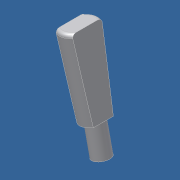
# Autodesk Inventor part: M20E-toggles
Saved by Autodesk Inventor 2015 SP1 (Build 190203100, 203)
## iProperties
Category: PARTsolutions
Created: 2013-12-29
Part Number: M20E-toggles
Catalog Web Link: www.cadenas.de
Description: Bushing Mount Miniature Toggles - toggles - Series M - Miniature Toggles
Document SubType Name: Modeling
Designer: PARTsolutions
Material: Generic
Density: 1 g/cm^3
Appearance: RGB(192,192,192)
NB: M20E-toggles
NN: Bushing Mount Miniature Toggles - toggles
NT: Series M - Miniature Toggles
NBSYN: $PN.-toggles
LINA: M20E-toggles
PN: M20E
SRS: M20
TGGLSALG: 'S', 'S - .413" (10.5mm) Bat','S2', 'S2 - .200" (5.08mm) Bat','S3', 'S3 - .256" (6.5mm) Bat','E', 'E - .450" (11.4mm) Flatted','E2', 'E2 - .256" (6.5mm) Flatted','E4', 'E4 - .840" (21.3mm) Flatted','Q', 'Q - .550" (14.0mm) Cone','Q2', 'Q2 - .640" (16.26mm) Cone','Q4', 'Q4 - .840" (21.3mm) Cone','C', 'C - .571" (14.5mm) Color Tipped Cone','D', 'D - .840" (21.3mm) Color Tipped Cone','K1', 'K1 - .370" (9.4mm) Paddle','K2', 'K2 - .559" (14.2mm) Paddle','B', 'B - .453" (11.5mm) Large Bat','B2', 'B2 - .689" (17.5mm) Large Bat','R', 'R - .610" (15.5mm) Large Flatted','L', 'L - .201" (5.1mm) Dia. Locking Lever'
TGGLS: E
CPSALG: '','N/A'
CCLRALG: '','N/A'
HEIGHT: 0.450
SHEIGHT: 0.087
ROTALG: 0.350
CPCAP: 0.000
KT: DUMMY
SUPPLIER: NKKSWITCHES
ARTICLENO: M20E-toggles
BOMINFO: M20E-toggles
CREATOR: CADENAS GmbH
PSOL_IDENT_0: {$CADENAS_DATA\23d-libs\nkkswitches\toggle\m\parts\m_bt_toggle.prj},215 {VTYP=3D},{NB=M20E-toggles},
PSOL_IDENT_1: {LINA=M20E-toggles},{NN=Bushing Mount Miniature Toggles - toggles},{DATE=28.05.2013 12:02:29},{GEOMD
PSOL_IDENT_2: ATE=28.05.2013 14:02:00},{VERSION=},{LINEID=10},{LINESUBID=-1},{WBVAR=TGGLS,CPS,CCLR}  {NB=M20E-togg
PSOL_IDENT_3: les},{LINA=M20E-toggles},{KT=DUMMY},{PN=M20E},{SRS=M20},{TGGLSALG='S', 'S - .413\" (10.5mm) Bat','S2
PSOL_IDENT_4: ', 'S2 - .200\" (5.08mm) Bat','S3', 'S3 - .256\" (6.5mm) Bat','E', 'E - .450\" (11.4mm) Flatted','E2
PSOL_IDENT_5: ', 'E2 - .256\" (6.5mm) Flatted','E4', 'E4 - .840\" (21.3mm) Flatted','Q', 'Q - .550\" (14.0mm) Cone
PSOL_IDENT_6: ','Q2', 'Q2 - .640\" (16.26mm) Cone','Q4', 'Q4 - .840\" (21.3mm) Cone','C', 'C - .571\" (14.5mm) Col
PSOL_IDENT_7: or Tipped Cone','D', 'D - .840\" (21.3mm) Color Tipped Cone','K1', 'K1 - .370\" (9.4mm) Paddle','K2'
PSOL_IDENT_8: , 'K2 - .559\" (14.2mm) Paddle','B', 'B - .453\" (11.5mm) Large Bat','B2', 'B2 - .689\" (17.5mm) Lar
PSOL_IDENT_9: ge Bat','R', 'R - .610\" (15.5mm) Large Flatted','L', 'L - .201\" (5.1mm) Dia. Locking Lever'},{TGGL
PSOL_IDENT_10: S=E},{CPSALG='','N/A'},{CPS=},{CPSPN=},{CCLRALG='','N/A'},{CCLR=},{DSH=},{HEIGHT=0.45},{SHEIGHT=0.08
PSOL_IDENT_11: 75},{ROTALG=0.35},{CPCAP=0}
Title: M20E-toggles
Author: Cadenas PARTsolutions
Comments: Series M - Miniature Toggles
Autodesk Inventor part; units mm, degrees
sketch "Sketch_4" plane through (0, 0, 0) normal (0, 0, 1) x (1, 0, 0)
  line L0 (0.481037, -4.392318) -> (-2.965747, 11.155122)
  line L1 (-2.965747, 11.155122) -> (-0.981914, 11.594927)
  arc A0 (-0.376004, 11.20892) -> (-0.981914, 11.594927) centre (-0.871963, 11.098969) ccw
  line L2 (-0.376004, 11.20892) -> (1.437371, 0.372619)
  line L3 (1.437371, 0.372619) -> (0.758859, 0.222196)
  line L4 (0.758859, 0.222196) -> (1.720933, -4.11744)
  line L5 (1.720933, -4.11744) -> (0.481037, -4.392318)
  line L6 (0.481037, -4.392318) -> (-2.965747, 11.155122)
  constraints: 14 end point, 2 point on circle, 1 centre point
revolve "Revolution1" add sketch "Sketch_4" angle 360 about axis through (0.481037, -4.392318, 0) along (0.2164396, -0.976296, 0)
sketch "Sketch_5" plane through (0, 0, 0) normal (0, 0, 1) x (1, 0, 0)
  line L0 (-7.235192, 12.810279) -> (-2.688894, -7.696745)
  line L1 (-2.688894, -7.696745) -> (4.750481, -6.047475)
  line L2 (4.750481, -6.047475) -> (0.204184, 14.459548)
  line L3 (0.204184, 14.459548) -> (-7.235192, 12.810279)
  line L4 (-4.205643, 10.880243) -> (-0.758859, -4.667196)
  line L5 (-0.758859, -4.667196) -> (1.720933, -4.11744)
  line L6 (1.720933, -4.11744) -> (-1.725851, 11.43)
  line L7 (-1.725851, 11.43) -> (-4.205643, 10.880243)
  constraints: 16 end point
extrude "Extrusion1" cut sketch "Sketch_5" along normal mid plane 5.08
ref_plane "rot_XY" through (0, -2.2225, 0) normal (0, 0, 1) x (1, 0, 0)
ref_plane "rot_YZ" through (0, -2.2225, 0) normal (1, 0, 0) x (0, 1, 0)
ref_plane "rot_ZX" through (0, -2.2225, 0) normal (0, 1, 0) x (0, 0, 1)
ref_plane "to_cap_XY" through (0, -2.2225, 0) normal (0, 1, 0) x (1, 0, 0)
ref_plane "to_cap_YZ" through (0, -2.2225, 0) normal (1, 0, 0) x (0, 0, -1)
ref_plane "to_cap_ZX" through (0, -2.2225, 0) normal (0, 0, -1) x (0, 1, 0)
body "Solid1"
